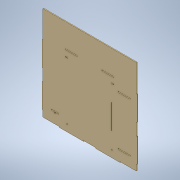
# Autodesk Inventor part: Base
Saved by Autodesk Inventor 2020 (Build 240168000, 168)
## iProperties
Created: 2020-03-09
Part Number: Base
Material: Genérico
Document SubType Name: Modeling
Designer: joser
Density: 1 g/cm^3
Appearance: Trigo
Author: joser
Autodesk Inventor part; units mm, degrees
ref_plane "YZ Plane" through (0, 0, 0) normal (1, 0, 0) x (0, 1, 0)
ref_plane "XZ Plane" through (0, 0, 0) normal (0, 1, 0) x (-1, 0, 0)
ref_plane "XY Plane" through (0, 0, 0) normal (0, 0, 1) x (1, 0, 0)
sketch "Boceto1" plane through (0, 0, 0) normal (0, 1, 0) x (-1, 0, 0)
  line L0 (-192, 193.5) -> (192, -193.5) construction
  line L1 (192, 193.5) -> (-192, -193.5) construction
  line L2 (-192, -168.5) -> (-195, -168.5)
  line L3 (-195, -168.5) -> (-195, -68.5)
  line L4 (-195, -68.5) -> (-192, -68.5)
  line L5 (-192, -193.5) -> (-192, -168.5)
  line L6 (-192, -18.5) -> (-195, -18.5)
  line L7 (-195, -18.5) -> (-195, 81.5)
  line L8 (-195, 81.5) -> (-192, 81.5)
  line L9 (-192, -68.5) -> (-192, -18.5)
  line L10 (-192, 81.5) -> (-192, 193.5)
  line L11 (100, 93.5) -> (50, 93.5)
  line L12 (50, 93.5) -> (50, 96.5)
  line L13 (50, 96.5) -> (100, 96.5)
  line L14 (100, 96.5) -> (100, 93.5)
  line L15 (-50, 96.5) -> (-100, 96.5)
  line L16 (-100, 96.5) -> (-100, 93.5)
  line L17 (-100, 93.5) -> (-50, 93.5)
  line L18 (-50, 93.5) -> (-50, 96.5)
  line L19 (-125, -193.5) -> (-125, -196.5)
  line L20 (-125, -196.5) -> (-25, -196.5)
  line L21 (-25, -196.5) -> (-25, -193.5)
  line L22 (25, -193.5) -> (25, -196.5)
  line L23 (25, -196.5) -> (125, -196.5)
  line L24 (125, -196.5) -> (125, -193.5)
  line L25 (-125, -193.5) -> (-192, -193.5)
  line L26 (192, -193.5) -> (125, -193.5)
  line L27 (25, -193.5) -> (-25, -193.5)
  line L28 (-192, 193.5) -> (192, 193.5)
  line L29 (192, -168.5) -> (195, -168.5)
  line L30 (195, -168.5) -> (195, -68.5)
  line L31 (195, -68.5) -> (192, -68.5)
  line L32 (192, -18.5) -> (195, -18.5)
  line L33 (195, -18.5) -> (195, 81.5)
  line L34 (195, 81.5) -> (192, 81.5)
  line L35 (192, -168.5) -> (192, -193.5)
  line L36 (192, 193.5) -> (192, 81.5)
  line L37 (192, -18.5) -> (192, -68.5)
  point P0 (0, 0)
  dimension "d5" = 100
  dimension "d7" = 100
  dimension "d8" = 50
  dimension "d9" = 3
  dimension "d12" = 50
  dimension "d13" = 3
  dimension "d14" = 100
  dimension "d59" = 100
  dimension "d61" = 100
  dimension "d63" = 50
  dimension "d64" = 3
  dimension "d75" = 25
  dimension "d76" = 50
  dimension "d77" = 100
  dimension "d78" = 3
  dimension "d79" = 3
  dimension "d81" = 3
  dimension "d83" = 390
  dimension "d84" = 390
  dimension "d85" = 67
  constraints: 76 end point, 26 perpendicular, 18 parallel, 10 collinear, 5 horizontal, 4 point on line, 2 midpoint, 2 vertical
  measures "d5" distance of L2.end L3.end
  measures "d7" distance of L6.end L7.end
  measures "d8" distance of L12.end L13.end
  measures "d9" distance of L11.end L12.end
  measures "d12" distance of L17.end L16.end
  measures "d13" distance of L16.end L15.end
  measures "d14" distance between parallel lines of L12 L18
  measures "d59" distance of L19.end L20.end
  measures "d61" distance of L22.end L23.end
  measures "d63" distance between parallel lines of L22 L21
  measures "d64" distance between parallel lines of L25 L20
  measures "d75" distance between parallel lines of L25 L2
  measures "d76" distance between parallel lines of L6 L4
  measures "d77" distance between parallel lines of L28 L11
  measures "d78" distance between parallel lines of L5 L3
  measures "d79" distance of L29.start L29.end
  measures "d81" distance of L32.start L32.end
  measures "d83" distance between parallel lines of L28 L23
  measures "d84" distance between parallel lines of L3 L30
  measures "d85" distance between parallel lines of L24 L35
extrude "Extrusión2" add sketch "Boceto1" along normal blind 3
sketch "Boceto2" plane through (0, 3, 0) normal (0, 1, 0) x (1, 0, 0)
  line L0 (72, -93.5) -> (72, 193.5) construction
  line L1 (192, 193.5) -> (-192, 193.5) projected
  line L2 (50, -93.5) -> (100, -93.5) projected
  line L3 (72, 50) -> (192, 50) construction
  line L4 (192, 18.5) -> (192, 68.5) projected
  line L5 (117, 153) -> (167, 153)
  line L6 (167, 153) -> (167, 150)
  line L7 (167, 150) -> (117, 150)
  line L8 (117, 150) -> (117, 153)
  line L9 (117, -50) -> (167, -50)
  line L10 (167, -50) -> (167, -53)
  line L11 (167, -53) -> (117, -53)
  line L12 (117, -53) -> (117, -50)
  line L13 (89, 100) -> (92, 100)
  line L14 (92, 100) -> (92, 0)
  line L15 (92, 0) -> (89, 0)
  line L16 (89, 0) -> (89, 100)
  point P0 (0, 0)
  point P1 (92, 50)
  dimension "d18" = 120
  dimension "d19" = 50
  dimension "d20" = 3
  dimension "d21" = 50
  dimension "d22" = 3
  dimension "d23" = 100
  dimension "d24" = 100
  dimension "d25" = 25
  dimension "d26" = 3
  dimension "d27" = 100
  dimension "d28" = 28
  constraints: 28 end point, 6 parallel, 5 point on line, 4 horizontal, 3 perpendicular, 2 midpoint, 1 vertical
  measures "d18" distance between parallel lines of L4 L0
  measures "d19" distance of L6.end L7.end
  measures "d20" distance of L5.end L6.end
  measures "d21" distance of L10.end L11.end
  measures "d22" distance between parallel lines of L11 L9
  measures "d23" distance between parallel lines of L9 L3
  measures "d24" distance between parallel lines of L3 L7
  measures "d25" distance between parallel lines of L4 L10
  measures "d26" distance of L14.end L15.end
  measures "d27" distance of L13.end L14.end
  measures "d28" distance between parallel lines of L12 L16
extrude "Extrusión3" cut sketch "Boceto2" against normal blind 3
hole "Agujero1" at (92, 3, -168.5) direction (0, -1, 0) diameter 5 end through all
hole "Agujero2" at (-92, 3, -168.5) direction (0, -1, 0) diameter 5 end through all
sketch "Boceto3" plane through (0, 3, 0) normal (0, 1, 0) x (1, 0, 0)
  circle A0 centre (92, -68.5) radius 2.5
  circle A1 centre (-92, -68.5) radius 2.5
  line L0 (-192, 193.5) -> (-192, -193.5) projected
  line L1 (192, -193.5) -> (192, -81.5) projected
  line L2 (-100, -93.5) -> (-50, -93.5) projected
  line L3 (99.5, -70) -> (96.5, -70)
  line L4 (96.5, -70) -> (96.5, -67)
  line L5 (96.5, -67) -> (99.5, -67)
  line L6 (99.5, -67) -> (99.5, -70)
  line L7 (-96.5, -70) -> (-99.5, -70)
  line L8 (-99.5, -70) -> (-99.5, -67)
  line L9 (-99.5, -67) -> (-96.5, -67)
  line L10 (-96.5, -67) -> (-96.5, -70)
  point P0 (0, 0)
  point P1 (99.5, -68.5)
  point P2 (-96.5, -68.5)
  dimension "d49" = 5
  dimension "d50" = 5
  dimension "d51" = 100
  dimension "d52" = 25
  dimension "d54" = 100
  dimension "d98" = 3
  dimension "d99" = 3
  dimension "d101" = 4.5
  dimension "d102" = 3
  dimension "d103" = 3
  dimension "d105" = 4.5
  constraints: 16 end point, 4 parallel, 3 horizontal alignment, 2 centre point, 2 horizontal, 2 midpoint, 2 perpendicular
  measures "d49" diameter of A0
  measures "d50" diameter of A1
  measures "d51" distance from line of L0 A1.centre
  measures "d52" distance from line of L2 A1.centre
  measures "d54" distance from line of L1 A0.centre
  measures "d98" distance of L4.end L5.end
  measures "d99" distance of L3.end L4.end
  measures "d101" distance from line of A0.centre L4
  measures "d102" distance of L8.end L9.end
  measures "d103" distance of L7.end L8.end
  measures "d105" distance from line of A1.centre L10
extrude "Extrusión4" cut sketch "Boceto3" against normal blind 3
sketch "Boceto4" plane through (0, 3, 0) normal (0, 1, 0) x (1, 0, 0)
  line L0 (-127, 150.5) -> (-157, 150.5)
  line L1 (-157, 150.5) -> (-157, 147.5)
  line L2 (-157, 147.5) -> (-127, 147.5)
  line L3 (-127, 147.5) -> (-127, 150.5)
  line L4 (-192, 193.5) -> (-192, 168.5) projected
  line L5 (-127, -46.5) -> (-157, -46.5)
  line L6 (-157, -46.5) -> (-157, -49.5)
  line L7 (-157, -49.5) -> (-127, -49.5)
  line L8 (-127, -49.5) -> (-127, -46.5)
  line L9 (-125, 193.5) -> (-192, 193.5) projected
  line L10 (-139.5, 152.5) -> (-144.5, 152.5)
  line L11 (-144.5, 152.5) -> (-144.5, 155.5)
  line L12 (-144.5, 155.5) -> (-139.5, 155.5)
  line L13 (-139.5, 155.5) -> (-139.5, 152.5)
  point P0 (0, 0)
  point P1 (-142, 152.5)
  point P2 (-142, 150.5)
  dimension "d86" = 30
  dimension "d87" = 3
  dimension "d88" = 35
  dimension "d89" = 30
  dimension "d90" = 3
  dimension "d93" = 194
  dimension "d94" = 43
  dimension "d95" = 5
  dimension "d96" = 3
  dimension "d97" = 2
  constraints: 24 end point, 6 parallel, 3 horizontal, 3 perpendicular, 2 midpoint, 1 collinear, 1 vertical alignment
  measures "d86" distance of L2.end L1.end
  measures "d87" distance of L1.end L0.end
  measures "d88" distance between parallel lines of L4 L1
  measures "d89" distance of L7.end L6.end
  measures "d90" distance of L6.end L5.end
  measures "d93" distance between parallel lines of L5 L2
  measures "d94" distance between parallel lines of L9 L0
  measures "d95" distance of L11.end L12.end
  measures "d96" distance of L10.end L11.end
  measures "d97" distance between parallel lines of L0 L10
extrude "Extrusión5" cut sketch "Boceto4" against normal blind 3 contours L3 L2 L1 L0 | L10 L11 L12 L13
